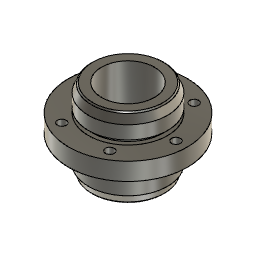
Model 21 (Autodesk Fusion 360 design; units mm, degrees)
Autodesk Fusion 360 part; units mm, degrees
sketch "Sketch1" plane through (0, 0, 0) normal (0, 0, 1) x (1, 0, 0)
  circle A0 centre (0, 0) radius 24
  circle A1 centre (0, 0) radius 36
  circle A2 centre (0, 0) radius 44 construction
  circle A3 centre (0, 0) radius 54
  line L0 (0, 0) -> (0, 54) construction
  line L1 (0, 0) -> (-26.6729, 46.9527) construction
  circle A4 centre (-21.7334, 38.2578) radius 4
  circle A5 centre (-43.9989, 0.3072) radius 4
  circle A6 centre (-22.2655, -37.9506) radius 4
  circle A7 centre (21.7334, -38.2578) radius 4
  circle A8 centre (43.9989, -0.3072) radius 4
  circle A9 centre (22.2655, 37.9506) radius 4
  dimension "d1" = 48
  dimension "d2" = 72
  dimension "d3" = 88
  dimension "d4" = 108
  dimension "d5" = 29.6
  dimension "d6" = 8
  dimension "d8" = 360
  constraint coincident A0.centre A1.centre
  constraint concentric A1 A2
  constraint concentric A0 A3
  constraint coincident A3 L0.end
  constraint vertical L0
  constraint coincident A3 L1.end
  constraint coincident A2 A4.centre
  constraint coincident L1 A4.centre
  measures "d1" diameter of A0
  measures "d2" diameter of A1
  measures "d3" diameter of A2
  measures "d4" diameter of A3
  measures "d5" angle of L0 L1
  measures "d6" diameter of A4
extrude "Extrude1" add sketch "Sketch1" along normal blind 72 contours A1 makes body 1
extrude "Extrude2" add sketch "Sketch1" along normal blind 16 from surface at 32 separate body contours A3 makes body 2
chamfer "Chamfer3" distance 4 angle 45 1 faces at (35.9552, -1.7945, 48) on bodies 1
chamfer "Chamfer4" distance 4 angle 45 1 faces at (35.8211, -3.5844, 46.6667) on bodies 1
sketch "Sketch2" plane through (0, 0, 0) normal (0, 1, 0) x (1, 0, 0)
  line L0 (-36, -32) -> (-36, 0)
  line L1 (-36, 0) -> (37, 0)
  line L2 (37, 0) -> (36.5, -33)
  line L3 (36.5, -33) -> (-36, -32)
  line L4 (-36, -32) -> (-41, -32)
  line L5 (36.5, -33) -> (41.5, -33)
  arc A0 (-32.0004, -32.0552) -> (-40, -32) centre (-36, -32) ccw
  line L6 (-36, -32) -> (-36, -48)
  line L7 (-36, -48) -> (36, -48)
  line L8 (-36, -48) -> (-43, -48)
  arc A1 (-40, -48) -> (-32, -48) centre (-36, -48) ccw
  dimension "d20" = 5
  dimension "d22" = 8
  dimension "d23" = 8
  constraint vertical L0
  constraint perpendicular L0 L1
  constraint perpendicular L0 L4
  constraint horizontal L5
  constraint coincident L0.start L3.end
  constraint coincident L4 A0.end
  constraint coincident L3 A0.start
  constraint perpendicular L4 L6
  constraint perpendicular L6 L7
  constraint perpendicular L6 L8
  constraint coincident L6.end L7.start
  constraint coincident L8 A1.start
  constraint coincident L7 A1.end
  measures "d20" distance of L2.end L5.end
  measures "d22" diameter of A0
  measures "d23" diameter of A1
revolve "Revolve2" cut sketch "Sketch2" angle 360 about axis through (0, 0, 0) along (0, 0, -1) contours L7 L8 A1 bodies 1
revolve "Revolve3" cut sketch "Sketch2" angle 360 about axis through (0, 0, 0) along (0, 0, -1) contours L0 L4 A0 | L0 L3 A0 bodies 1
equation "d9 = 32 mm + 16 mm + 24 mm"
